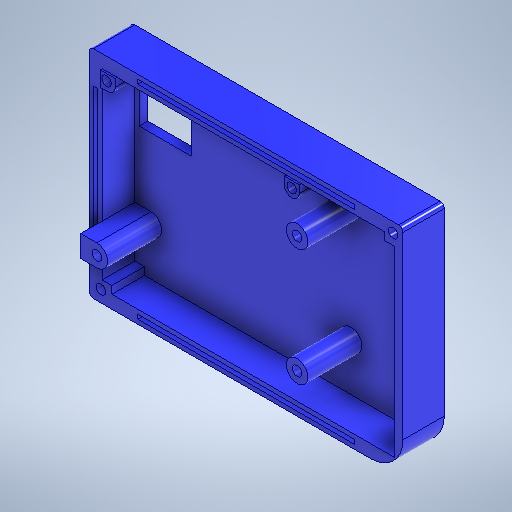
# Autodesk Inventor part: Krabicka_dolni
Saved by Autodesk Inventor 2025.2 (Build 292293000, 293)
## iProperties
Created: 2025-03-24
Part Number: Krabicka_dolni
Material: Všeobecné
Document SubType Name: Modeling
Designer: jakub
Density: 1 g/cm^3
Appearance: Modrá – nástěnná malba – lesklá
Author: jakub
## iProperties of the stored document Krabicka_dolni_3D tisk.ipt
Created: 2025-03-26
Part Number: Krabicka_dolni_3D tisk
Material: Všeobecné
Document SubType Name: Modeling
Designer: jakub
Density: 1 g/cm^3
Appearance: Výchozí
Author: jakub
Autodesk Inventor part; units mm, degrees
ref_plane "YZ Plane" through (0, 0, 0) normal (1, 0, 0) x (0, 1, 0)
ref_plane "XZ Plane" through (0, 0, 0) normal (0, 1, 0) x (-1, 0, 0)
ref_plane "XY Plane" through (0, 0, 0) normal (0, 0, 1) x (1, 0, 0)
sketch "Náčrt1" plane through (0, 0, 0) normal (0, 0, 1) x (1, 0, 0)
  line L0 (0, 71.6213) -> (0, -79.7279) projected
  line L1 (-102.1213, 0) -> (105.2279, 0) projected
  line L2 (-72.5, 50) -> (72.5, 50)
  line L3 (72.5, 50) -> (72.5, -35)
  line L4 (57.5, -50) -> (-72.5, -50)
  line L5 (-72.5, -50) -> (-72.5, 50)
  arc A0 (57.5, -50) -> (72.5, -35) centre (57.5, -35) ccw
  point P0 (0, 0)
  point P1 (-72.5, 0)
  point P2 (0, -50)
  point P3 (0, 50)
  point P4 (72.5, 0)
  dimension "d0" = 130
  dimension "d1" = 100
  dimension "d2" = 30
  constraints: 8 end point, 2 parallel, 2 point on circle, 2 tangent, 1 centre point, 1 horizontal, 1 perpendicular, 2 other
  measures "d0" distance of L4.start L4.end
  measures "d1" distance between parallel lines of L4 L2
  measures "d2" diameter of A0
extrude "Vysunutí1" add sketch "Náčrt1" along normal blind 33
sketch "Náčrt2" plane through (0, 0, 33) normal (0, 0, 1) x (1, 0, 0)
  line L0 (-72.5, -50) -> (57.5, -50) projected
  arc A0 (57.5, -50) -> (72.5, -35) centre (57.5, -35) ccw projected
  line L1 (72.5, -35) -> (72.5, 50) projected
  line L2 (72.5, 50) -> (-72.5, 50) projected
  line L3 (-72.5, 50) -> (-72.5, -50) projected
  line L4 (-66.5, 44) -> (68.5, 44)
  line L5 (68.5, 44) -> (68.5, -31.5)
  line L6 (54, -44) -> (-66.5, -44)
  line L7 (-66.5, -44) -> (-66.5, 44)
  line L8 (54, -44) -> (68.5, -44)
  line L9 (68.5, -44) -> (68.5, -31.5)
  point P0 (0, 0)
  dimension "d5" = 4
  dimension "d6" = 6
  dimension "d7" = 6
  dimension "d8" = 6
  constraints: 12 end point, 2 horizontal, 2 parallel, 2 perpendicular
  measures "d5" distance between parallel lines of L5 L1
  measures "d6" distance between parallel lines of L0 L6
  measures "d7" distance between parallel lines of L3 L7
  measures "d8" distance between parallel lines of L4 L2
extrude "Vysunutí2" cut sketch "Náčrt2" against normal blind 29 contours L4 L5 L9 L8 L6 L7
fillet "Zaoblení1" radius 2 1 edges at (72.5, 50, 16.5)
fillet "Zaoblení2" radius 2 2 edges at (-72.5, 50, 16.5) (-72.5, -50, 16.5)
sketch "Náčrt3" plane through (0, 0, 4) normal (0, 0, 1) x (1, 0, 0)
  line L0 (68.5, 44) -> (68.5, -44) projected
  line L1 (-66.5, 44) -> (68.5, 44) projected
  line L2 (-66.5, -44) -> (-66.5, 44) projected
  line L3 (68.5, -44) -> (-66.5, -44) projected
  arc A0 (-72.5, -48) -> (-70.5, -50) centre (-70.5, -48) ccw projected
  line L4 (-70.5, -50) -> (57.5, -50) projected
  arc A1 (57.5, -50) -> (72.5, -35) centre (57.5, -35) ccw projected
  line L5 (72.5, -35) -> (72.5, 48) projected
  arc A2 (72.5, 48) -> (70.5, 50) centre (70.5, 48) ccw projected
  line L6 (70.5, 50) -> (-70.5, 50) projected
  arc A3 (-70.5, 50) -> (-72.5, 48) centre (-70.5, 48) ccw projected
  line L7 (-72.5, 48) -> (-72.5, -48) projected
  line L8 (-66.5, 44) -> (68.5, 44) projected
  line L9 (68.5, 44) -> (68.5, -44) projected
  line L10 (68.5, -44) -> (-66.5, -44) projected
  line L11 (-66.5, -44) -> (-66.5, 44) projected
  arc A4 (-63, 37) -> (-59.5, 40.5) centre (-63, 40.5) ccw
  line L12 (-66.5, 44) -> (68.5, 44) projected
  line L13 (-66.5, -44) -> (-66.5, 44) projected
  line L14 (-59.5, 40.5) -> (-59.5, 44)
  line L15 (-63, 37) -> (-66.5, 37)
  arc A5 (18.5, 40.5) -> (25.5, 40.5) centre (22, 40.5) ccw
  line L16 (25.5, 40.5) -> (25.5, 44)
  line L17 (18.5, 40.5) -> (18.5, 44)
  circle A6 centre (33.5, 32) radius 5
  circle A7 centre (20.5, -20.4118) radius 5
  arc A8 (-58.5, 21.7369) -> (-58.5, 31.7369) centre (-58.5, 26.7369) ccw
  line L18 (-58.5, 31.7369) -> (-66.5, 31.7369)
  line L19 (-58.5, 21.7369) -> (-66.5, 21.7369)
  point P0 (0, 0)
  point P1 (25.5, 42.25)
  point P2 (25.5, 44)
  point P3 (18.5, 44)
  point P4 (-66.5, 37)
  dimension "d14" = 7
  dimension "d15" = 7
  dimension "d16" = 85
  dimension "d17" = 10
  dimension "d18" = 8
  dimension "d19" = 8.5
  dimension "d20" = 10
  dimension "d21" = 54
  dimension "d22" = 48
  dimension "d23" = 10
  dimension "d24" = 92
  dimension "d25" = 8
  constraints: 12 end point, 9 tangent, 6 perpendicular, 6 point on circle, 6 point on line, 5 centre point, 1 midpoint
  measures "d14" diameter of A4
  measures "d15" diameter of A5
  measures "d16" distance of A4.centre A5.centre
  measures "d17" diameter of A6
  measures "d18" horizontal distance of point (25.5, 42.25) A6.centre
  measures "d19" vertical distance of A5.centre A6.centre
  measures "d20" diameter of A7
  measures "d21" distance of A7.centre A6.centre
  measures "d22" distance from line of L0 A7.centre
  measures "d23" diameter of A8
  measures "d24" distance of A8.centre A7.centre
  measures "d25" distance of L18.start L18.end
extrude "Vysunutí3" add sketch "Náčrt3" along normal blind 16 contours L16 A5 L17 L1 | L14 A4 L15 L2 L1
sketch "Náčrt4" plane through (0, 0, 4) normal (0, 0, 1) x (1, 0, 0)
  line L0 (25.5, 44) -> (25.5, 40.5) projected
  arc A0 (18.5, 40.5) -> (25.5, 40.5) centre (22, 40.5) ccw projected
  line L1 (18.5, 40.5) -> (18.5, 44) projected
  line L2 (-59.5, 44) -> (18.5, 44) projected
  line L3 (-59.5, 44) -> (-59.5, 40.5) projected
  arc A1 (-63, 37) -> (-59.5, 40.5) centre (-63, 40.5) ccw projected
  line L4 (-63, 37) -> (-66.5, 37) projected
  line L5 (-66.5, -44) -> (-66.5, 37) projected
  line L6 (68.5, -44) -> (-66.5, -44) projected
  line L7 (68.5, 44) -> (68.5, -44) projected
  line L8 (25.5, 44) -> (68.5, 44) projected
  circle A2 centre (33.5, 32) radius 5
  circle A3 centre (33.5, -22) radius 5
  circle A4 centre (-59, -22) radius 5
  line L9 (-59, -17) -> (-66.5, -17)
  line L10 (-59, -27) -> (-66.5, -27)
  point P0 (0, 0)
  dimension "d28" = 10
  dimension "d29" = 10
  dimension "d30" = 10
  dimension "d31" = 8
  dimension "d32" = 8.5
  dimension "d33" = 54
  dimension "d61" = 92.5
  dimension "d62" = 7.5
  dimension "d77" = 100
  constraints: 4 end point, 3 centre point, 2 perpendicular, 2 point on circle, 2 point on line, 2 tangent
  measures "d28" diameter of A2
  measures "d29" diameter of A3
  measures "d30" diameter of A4
  measures "d31" distance from line of L0 A2.centre
  measures "d32" vertical distance of A0.centre A2.centre
  measures "d33" distance of A3.centre A2.centre
  measures "d61" distance of A3.centre A4.centre
  measures "d62" distance of L9.start L9.end
  measures "d77" distance from line of L5 A3.centre
extrude "Vysunutí4" add sketch "Náčrt4" along normal blind 25 contours L5 L9 A4 L10 | A4 | A2 | A3
sketch "Náčrt6" plane through (0, 0, 4) normal (0, 0, 1) x (1, 0, 0)
  line L0 (-64.5, 30.5) -> (-40.5, 30.5)
  line L1 (-40.5, 30.5) -> (-40.5, 14.5)
  line L2 (-40.5, 14.5) -> (-64.5, 14.5)
  line L3 (-64.5, 14.5) -> (-64.5, 30.5)
  line L4 (-66.5, 44) -> (68.5, 44) projected
  line L5 (-66.5, -44) -> (-66.5, 44) projected
  point P0 (0, 0)
  dimension "d41" = 24
  dimension "d42" = 16
  dimension "d43" = 13.5
  dimension "d44" = 2
  constraints: 8 end point, 2 parallel, 1 horizontal, 1 perpendicular
  measures "d41" distance of L1.end L2.end
  measures "d42" distance of L0.end L1.end
  measures "d43" distance between parallel lines of L4 L0
  measures "d44" distance between parallel lines of L5 L3
extrude "Vysunutí5" cut sketch "Náčrt6" against normal blind 33
sketch "Náčrt8" plane through (0, 0, 33) normal (0, 0, 1) x (1, 0, 0)
  arc A0 (-72.5, -48) -> (-70.5, -50) centre (-70.5, -48) ccw projected
  line L0 (-70.5, -50) -> (57.5, -50) projected
  arc A1 (57.5, -50) -> (72.5, -35) centre (57.5, -35) ccw projected
  line L1 (72.5, -35) -> (72.5, 48) projected
  arc A2 (72.5, 48) -> (70.5, 50) centre (70.5, 48) ccw projected
  line L2 (70.5, 50) -> (-70.5, 50) projected
  arc A3 (-70.5, 50) -> (-72.5, 48) centre (-70.5, 48) ccw projected
  line L3 (-72.5, 48) -> (-72.5, -48) projected
  line L4 (-66.5, 44) -> (68.5, 44) projected
  line L5 (68.5, 44) -> (68.5, -44) projected
  line L6 (68.5, -44) -> (-66.5, -44) projected
  line L7 (-66.5, -44) -> (-66.5, 44) projected
  line L8 (-66.5, 44) -> (68.5, 44)
  line L9 (68.5, 44) -> (68.5, -44)
  line L10 (68.5, -44) -> (-66.5, -44)
  line L11 (-66.5, -44) -> (-66.5, 44)
  arc A4 (57.5, -50) -> (72.5, -35) centre (57.5, -35) ccw
  line L12 (72.5, -35) -> (72.5, 48.1384)
  line L13 (70.5, 50) -> (-70.5, 50)
  line L14 (-72.5, 48) -> (-72.5, -48)
  line L15 (-70.5, -50) -> (57.5, -50)
  circle A5 centre (-70.5, -48) radius 2
  circle A6 centre (-70.5, 48) radius 2
  circle A7 centre (70.5, 48) radius 2
  point P0 (0, 0)
  constraints: 16 end point, 4 centre point, 4 coincident, 4 concentric, 4 point on line, 3 equal length, 2 point on circle, 1 horizontal, 1 perpendicular
extrude "Vysunutí6" cut sketch "Náčrt8" against normal blind 13.9
sketch "Náčrt9" plane through (0, 0, 20) normal (0, 0, 1) x (1, 0, 0)
  line L0 (-59.5, 40.5) -> (-59.5, 44) projected
  line L1 (-66.5, 44) -> (-59.5, 44) projected
  line L2 (-66.5, 37) -> (-66.5, 44) projected
  line L3 (-66.5, 37) -> (-63, 37) projected
  arc A0 (-63, 37) -> (-59.5, 40.5) centre (-63, 40.5) ccw projected
  line L4 (25.5, 40.5) -> (25.5, 44) projected
  line L5 (18.5, 44) -> (25.5, 44) projected
  line L6 (18.5, 44) -> (18.5, 40.5) projected
  arc A1 (18.5, 40.5) -> (25.5, 40.5) centre (22, 40.5) ccw projected
  circle A2 centre (-63.5, 41) radius 2.2
  circle A3 centre (22, 41) radius 2.2
  point P0 (0, 0)
  dimension "d49" = 4.4
  dimension "d50" = 3
  dimension "d51" = 3
  dimension "d52" = 4.4
  dimension "d53" = 3
  dimension "d54" = 3.5
  constraints: 2 centre point
  measures "d49" diameter of A2
  measures "d50" distance from line of L1 A2.centre
  measures "d51" distance from line of L2 A2.centre
  measures "d52" diameter of A3
  measures "d53" distance from line of L5 A3.centre
  measures "d54" distance from line of L6 A3.centre
extrude "Vysunutí7" cut sketch "Náčrt9" against normal blind 8 contours A2 | A3
sketch "Náčrt10" plane through (33.5, 32, 29) normal (0, 0, 1) x (1, 0, 0)
  circle A0 centre (0, 0) radius 5 projected
  circle A1 centre (0, -54) radius 5 projected
  line L0 (-92.5, -49) -> (-100, -49) projected
  line L1 (-100, -59) -> (-100, -49) projected
  line L2 (-100, -59) -> (-92.5, -59) projected
  arc A2 (-92.5, -59) -> (-92.5, -49) centre (-92.5, -54) ccw projected
  circle A3 centre (0, 0) radius 2.2
  circle A4 centre (0, -54) radius 2.2
  point P0 (-33.5, -32)
  dimension "d57" = 4.4
  dimension "d58" = 4.4
  constraints: 2 centre point, 2 coincident
  measures "d57" diameter of A3
  measures "d58" diameter of A4
extrude "Vysunutí8" cut sketch "Náčrt10" against normal blind 8 contours A3 | A4
sketch "Náčrt11" plane through (0, 0, 29) normal (0, 0, 1) x (1, 0, 0)
  line L0 (-59, -17) -> (-66.5, -17) projected
  line L1 (-66.5, -27) -> (-66.5, -17) projected
  line L2 (-66.5, -27) -> (-59, -27) projected
  arc A0 (-59, -27) -> (-59, -17) centre (-59, -22) ccw projected
  circle A1 centre (-59, -22) radius 2.2
  point P0 (0, 0)
  dimension "d63" = 4.4
  constraints: 1 centre point, 1 coincident
  measures "d63" diameter of A1
extrude "Vysunutí9" cut sketch "Náčrt11" against normal blind 8 contours A1
sketch "Náčrt12" plane through (0, 0, 20) normal (0, 0, 1) x (1, 0, 0)
  line L0 (-66.5, 37) -> (-63, 37) projected
  circle A0 centre (-63.5, 41) radius 2.2 projected
  line L1 (-59.5, 40.5) -> (-59.5, 44) projected
  line L2 (-66.5, 44) -> (-59.5, 44) projected
  line L3 (-66.5, 37) -> (-66.5, 44) projected
  line L4 (-66.5, 37) -> (-63, 37) projected
  arc A1 (-63, 37) -> (-59.5, 40.5) centre (-63, 40.5) ccw projected
  circle A2 centre (22, 41) radius 2.2 projected
  line L5 (25.5, 40.5) -> (25.5, 44) projected
  line L6 (18.5, 44) -> (25.5, 44) projected
  line L7 (18.5, 44) -> (18.5, 40.5) projected
  arc A3 (18.5, 40.5) -> (25.5, 40.5) centre (22, 40.5) ccw projected
  line L8 (-65.9036, 43.7615) -> (24.0964, 43.7615) construction
  line L9 (24.0964, 43.7615) -> (24.0964, -3.2385) construction
  line L10 (24.0964, -3.2385) -> (-65.9036, -3.2385) construction
  line L11 (-65.9036, -3.2385) -> (-65.9036, 43.7615) construction
  point P0 (0, 0)
  dimension "d66" = 90
  dimension "d67" = 47
  constraints: 8 end point, 2 parallel, 1 horizontal, 1 perpendicular
  measures "d66" distance of L9.end L10.end
  measures "d67" distance of L8.end L9.end
sketch "Náčrt13" plane through (0, 0, 29) normal (0, 0, 1) x (1, 0, 0)
  circle A0 centre (-59, -22) radius 2.2 projected
  line L0 (-59, -17) -> (-66.5, -17) projected
  line L1 (-66.5, -27) -> (-66.5, -17) projected
  line L2 (-66.5, -27) -> (-59, -27) projected
  arc A1 (-59, -27) -> (-59, -17) centre (-59, -22) ccw projected
  circle A2 centre (33.5, -22) radius 2.2 projected
  circle A3 centre (33.5, -22) radius 5 projected
  circle A4 centre (33.5, 32) radius 5 projected
  circle A5 centre (33.5, 32) radius 2.2 projected
  line L3 (-62.1019, -25.0857) -> (36.3981, -25.0857) construction
  line L4 (36.3981, -25.0857) -> (36.3981, 34.9143) construction
  line L5 (36.3981, 34.9143) -> (-62.1019, 34.9143) construction
  line L6 (-62.1019, 34.9143) -> (-62.1019, -25.0857) construction
  point P0 (0, 0)
  dimension "d68" = 98.5
  dimension "d69" = 60
  constraints: 8 end point, 2 parallel, 1 horizontal, 1 perpendicular
  measures "d68" distance of L5.end L4.end
  measures "d69" distance of L4.end L3.end
sketch "Náčrt15" plane through (0, 0, 4) normal (0, 0, 1) x (1, 0, 0)
  line L0 (-70.5, 50) -> (70.5, 50) projected
  arc A0 (-70.5, 50) -> (-72.5, 48) centre (-70.5, 48) ccw projected
  line L1 (-72.5, -48) -> (-72.5, 48) projected
  arc A1 (-72.5, -48) -> (-70.5, -50) centre (-70.5, -48) ccw projected
  line L2 (57.5, -50) -> (-70.5, -50) projected
  arc A2 (57.5, -50) -> (72.5, -35) centre (57.5, -35) ccw projected
  line L3 (72.5, 48) -> (72.5, -35) projected
  arc A3 (72.5, 48) -> (70.5, 50) centre (70.5, 48) ccw projected
  line L4 (-66.5, 37) -> (-66.5, -17) projected
  line L5 (18.5, 44) -> (-59.5, 44) projected
  line L6 (68.5, -44) -> (68.5, 44) projected
  line L7 (-66.5, -44) -> (68.5, -44) projected
  line L8 (-66.5, -27) -> (-66.5, -44) projected
  line L9 (-66.5, -17) -> (-66.5, -27) projected
  line L10 (-66.5, 44) -> (-66.5, 37) projected
  line L11 (-59.5, 44) -> (-66.5, 44) projected
  line L12 (25.5, 44) -> (18.5, 44) projected
  line L13 (68.5, 44) -> (25.5, 44) projected
  point P0 (0, 0)
sketch "Náčrt16" plane through (0, 0, 4) normal (0, 0, 1) x (1, 0, 0)
  line L0 (68.5, -44) -> (-66.5, -44) projected
  line L1 (68.5, 44) -> (68.5, -44) projected
  line L2 (41.5, -44) -> (68.5, -44)
  line L3 (68.5, -44) -> (68.5, -40)
  arc A0 (57.5, -50) -> (72.5, -35) centre (57.5, -35) ccw construction
  point P0 (0, 0)
  point P1 (68.5, -23.5)
  point P2 (68.5, -30.5)
  constraints: 4 end point, 4 point on line, 1 horizontal, 1 perpendicular
extrude "Vysunutí10" [suppressed]
sketch "Náčrt17" plane through (47, -27, 6) normal (0, 0, 1) x (1, 0, 0)
  circle A0 centre (0, 0) radius 3.5 projected
  line L0 (-117.5, 77) -> (23.5, 77) projected
  arc A1 (-117.5, 77) -> (-119.5, 75) centre (-117.5, 75) ccw projected
  line L1 (-119.5, -21) -> (-119.5, 75) projected
  arc A2 (-119.5, -21) -> (-117.5, -23) centre (-117.5, -21) ccw projected
  line L2 (10.5, -23) -> (-117.5, -23) projected
  arc A3 (10.5, -23) -> (25.5, -8) centre (10.5, -8) ccw projected
  line L3 (25.5, 75) -> (25.5, -8) projected
  arc A4 (25.5, 75) -> (23.5, 77) centre (23.5, 75) ccw projected
  line L4 (-113.5, 64) -> (-113.5, 10) projected
  line L5 (-28.5, 71) -> (-106.5, 71) projected
  line L6 (21.5, -17) -> (21.5, 71) projected
  line L7 (-113.5, -17) -> (21.5, -17) projected
  line L8 (17, -3.5) -> (21.5, -3.5) projected
  line L9 (21.5, 3.5) -> (21.5, -3.5) projected
  line L10 (21.5, 3.5) -> (17, 3.5) projected
  arc A5 (17, 3.5) -> (17, -3.5) centre (17, 0) ccw projected
  line L11 (21.5, 3.5) -> (21.5, -3.5) projected
  line L12 (-113.5, 0) -> (-113.5, -17) projected
  line L13 (-113.5, 10) -> (-113.5, 0) projected
  line L14 (-113.5, 71) -> (-113.5, 64) projected
  line L15 (-106.5, 71) -> (-113.5, 71) projected
  line L16 (-21.5, 71) -> (-28.5, 71) projected
  line L17 (21.5, 71) -> (-21.5, 71) projected
  line L18 (17, -3.5) -> (21.5, -3.5) projected
  line L19 (21.5, 3.5) -> (17, 3.5) projected
  arc A6 (17, 3.5) -> (17, -3.5) centre (17, 0) ccw projected
  point P0 (-47, 27)
  constraints: 2 coincident
hole "Díra1" [suppressed]
sketch "Náčrt19" plane through (33.5, -22, 29) normal (0, 0, 1) x (1, 0, 0)
  point P0 (-33.5, 22)
sketch "Náčrt20" plane through (0, 0, 19.1) normal (0, 0, 1) x (1, 0, 0)
  line L0 (-70.5, 50) -> (70.5, 50) projected
  arc A0 (-70.5, 50) -> (-72.5, 48) centre (-70.5, 48) ccw projected
  line L1 (-72.5, -48) -> (-72.5, 48) projected
  arc A1 (-72.5, -48) -> (-70.5, -50) centre (-70.5, -48) ccw projected
  line L2 (57.5, -50) -> (-70.5, -50) projected
  arc A2 (57.5, -50) -> (72.5, -35) centre (57.5, -35) ccw projected
  line L3 (72.5, 48) -> (72.5, -35) projected
  arc A3 (72.5, 48) -> (70.5, 50) centre (70.5, 48) ccw projected
  line L4 (-66.5, 37) -> (-66.5, -17) projected
  line L5 (18.5, 44) -> (-59.5, 44) projected
  line L6 (68.5, -44) -> (68.5, 44) projected
  line L7 (-66.5, -44) -> (68.5, -44) projected
  line L8 (-50, 48) -> (50, 48)
  line L9 (50, 48) -> (50, 46)
  line L10 (50, 46) -> (-50, 46)
  line L11 (-50, 46) -> (-50, 48)
  line L12 (0, 71.1184) -> (0, -73.8108) projected
  line L13 (-102.6184, 0) -> (105.3108, 0) projected
  line L14 (-50, -48) -> (50, -48)
  line L15 (50, -48) -> (50, -46)
  line L16 (50, -46) -> (-50, -46)
  line L17 (-50, -46) -> (-50, -48)
  line L18 (-70.5, 35) -> (-68.5, 35)
  line L19 (-68.5, 35) -> (-68.5, -35)
  line L20 (-68.5, -35) -> (-70.5, -35)
  line L21 (-70.5, -35) -> (-70.5, 35)
  line L22 (-66.5, -27) -> (-66.5, -44) projected
  line L23 (-66.5, -17) -> (-66.5, -27) projected
  line L24 (-66.5, 44) -> (-66.5, 37) projected
  line L25 (-59.5, 44) -> (-66.5, 44) projected
  line L26 (25.5, 44) -> (18.5, 44) projected
  line L27 (68.5, 44) -> (25.5, 44) projected
  point P0 (0, 0)
  dimension "d103" = 100
  dimension "d104" = 2
  dimension "d105" = 2
  dimension "d106" = 2
  dimension "d107" = 70
  dimension "d108" = 2
  constraints: 24 end point, 4 parallel, 4 symmetric about line, 2 horizontal, 2 perpendicular, 2 other
  measures "d103" distance of L9.end L10.end
  measures "d104" distance of L8.end L9.end
  measures "d105" distance between parallel lines of L0 L8
  measures "d106" distance of L19.end L20.end
  measures "d107" distance of L18.end L19.end
  measures "d108" distance between parallel lines of L4 L19
extrude "Vysunutí11" cut sketch "Náčrt20" against normal blind 10 contours L12 L10 L11 L8 | L8 L9 L10 L12 | L21 L18 L19 L13 | L13 L19 L20 L21 | L14 L17 L16 L12 | L12 L16 L15 L14
sketch "Náčrt22" plane through (0, 0, 4) normal (0, 0, 1) x (1, 0, 0)
  line L0 (50, -46) -> (50, -48) projected
  line L1 (50, -48) -> (-50, -48) projected
  line L2 (-50, -48) -> (-50, -46) projected
  line L3 (-50, -46) -> (50, -46) projected
  line L4 (-70.5, 35) -> (-68.5, 35) projected
  line L5 (-68.5, 35) -> (-68.5, -35) projected
  line L6 (-68.5, -35) -> (-70.5, -35) projected
  line L7 (-70.5, -35) -> (-70.5, 35) projected
  line L8 (-50, 46) -> (-50, 48) projected
  line L9 (-50, 48) -> (50, 48) projected
  line L10 (50, 48) -> (50, 46) projected
  line L11 (50, 46) -> (-50, 46) projected
  line L12 (-70.5, 50) -> (70.5, 50) projected
  arc A0 (-70.5, 50) -> (-72.5, 48) centre (-70.5, 48) ccw projected
  line L13 (-72.5, -48) -> (-72.5, 48) projected
  arc A1 (-72.5, -48) -> (-70.5, -50) centre (-70.5, -48) ccw projected
  line L14 (57.5, -50) -> (-70.5, -50) projected
  arc A2 (57.5, -50) -> (72.5, -35) centre (57.5, -35) ccw projected
  line L15 (72.5, 48) -> (72.5, -35) projected
  arc A3 (72.5, 48) -> (70.5, 50) centre (70.5, 48) ccw projected
  line L16 (-66.5, 44) -> (-66.5, 37) projected
  line L17 (-59.5, 44) -> (-66.5, 44) projected
  line L18 (18.5, 44) -> (-59.5, 44) projected
  line L19 (25.5, 44) -> (18.5, 44) projected
  line L20 (68.5, 44) -> (25.5, 44) projected
  line L21 (68.5, -44) -> (68.5, 44) projected
  line L22 (-66.5, -44) -> (68.5, -44) projected
  line L23 (-66.5, -27) -> (-66.5, -44) projected
  line L24 (-66.5, -17) -> (-66.5, -27) projected
  line L25 (-66.5, 37) -> (-66.5, -17) projected
  circle A4 centre (33.5, 32) radius 5 projected
  circle A5 centre (33.5, -22) radius 5 projected
  line L26 (68.5, 44) -> (68.5, -44) projected
  line L27 (25.5, 44) -> (68.5, 44) projected
  line L28 (25.5, 44) -> (25.5, 40.5) projected
  arc A6 (18.5, 40.5) -> (25.5, 40.5) centre (22, 40.5) ccw projected
  line L29 (18.5, 40.5) -> (18.5, 44) projected
  line L30 (-59.5, 44) -> (18.5, 44) projected
  line L31 (-59.5, 44) -> (-59.5, 40.5) projected
  arc A7 (-63, 37) -> (-59.5, 40.5) centre (-63, 40.5) ccw projected
  line L32 (-63, 37) -> (-66.5, 37) projected
  line L33 (-66.5, -17) -> (-66.5, 37) projected
  line L34 (-66.5, -17) -> (-59, -17) projected
  arc A8 (-59, -27) -> (-59, -17) centre (-59, -22) ccw projected
  line L35 (-59, -27) -> (-66.5, -27) projected
  line L36 (-66.5, -44) -> (-66.5, -27) projected
  line L37 (68.5, -44) -> (-66.5, -44) projected
  line L38 (-40.5, 30.5) -> (-40.5, 14.5) projected
  line L39 (-40.5, 14.5) -> (-64.5, 14.5) projected
  line L40 (-64.5, 14.5) -> (-64.5, 30.5) projected
  line L41 (-64.5, 30.5) -> (-40.5, 30.5) projected
  line L42 (68.5, 44) -> (64, 44)
  line L43 (64, 44) -> (64, 40.5)
  line L44 (64, 40.5) -> (68.5, 40.5)
  line L45 (68.5, 40.5) -> (68.5, 44)
  line L46 (-66.5, -44) -> (-66.5, -27) projected
  line L47 (-66.5, -44) -> (-62, -44)
  line L48 (-62, -44) -> (-62, -40.5)
  line L49 (-62, -40.5) -> (-66.5, -40.5)
  line L50 (-66.5, -40.5) -> (-66.5, -44)
  point P0 (0, 0)
  dimension "d119" = 4.5
  dimension "d120" = 3.5
  dimension "d121" = 4.5
  dimension "d122" = 3.5
  constraints: 16 end point, 4 parallel, 2 horizontal, 2 perpendicular
  measures "d119" distance of L43.end L44.end
  measures "d120" distance of L42.end L43.end
  measures "d121" distance of L49.end L48.end
  measures "d122" distance of L48.end L47.end
extrude "Vysunutí13" add sketch "Náčrt22" along normal up to surface (15.1 mm away) contours L49 L48 L22 L23 | L20 L21 L44 L43
sketch "Náčrt23" plane through (0, 0, 19.1) normal (0, 0, 1) x (1, 0, 0)
  circle A0 centre (-67, -44.5) radius 2.2
  line L0 (57.5, -50) -> (-70.5, -50) projected
  line L1 (-72.5, -48) -> (-72.5, 48) projected
  circle A1 centre (68, 45.5) radius 2.2
  line L2 (72.5, 48) -> (72.5, -35) projected
  line L3 (-70.5, 50) -> (70.5, 50) projected
  point P0 (0, 0)
  dimension "d125" = 4.4
  dimension "d126" = 5.5
  dimension "d127" = 5.5
  dimension "d128" = 4.4
  dimension "d129" = 4.5
  dimension "d130" = 4.5
  constraints: 2 centre point
  measures "d125" diameter of A0
  measures "d126" distance from line of L0 A0.centre
  measures "d127" distance from line of L1 A0.centre
  measures "d128" diameter of A1
  measures "d129" distance from line of L2 A1.centre
  measures "d130" distance from line of L3 A1.centre
extrude "Vysunutí14" cut sketch "Náčrt23" against normal blind 8
sketch "Náčrt24" plane through (47, -27, 3) normal (0, 0, 1) x (1, 0, 0)
  point P0 (-47, 27)
